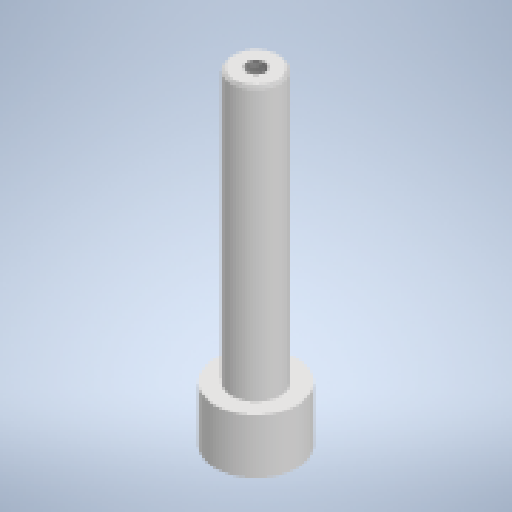
# Autodesk Inventor part: приводной вал
Saved by Autodesk Inventor 2023.2 (Build 272271030, 271C)
## iProperties
Created: 2023-08-07
Part Number: приводной вал
Material: Generic
Document SubType Name: Modeling
Designer: admin
Density: 1 g/cm^3
Appearance: Default
Author: admin
Autodesk Inventor part; units mm, degrees
ref_plane "XZ Plane" through (0, 0, 0) normal (0, 1, 0) x (-1, 0, 0)
ref_plane "XY Plane" through (0, 0, 0) normal (0, 0, 1) x (1, 0, 0)
sketch "Sketch1" plane through (0, 0, 0) normal (0, 0, 1) x (1, 0, 0)
  line L0 (0, 60) -> (0, -60)
  line L1 (0, -60) -> (15, -60)
  line L2 (9, 60) -> (0, 60)
  line L3 (9, -40) -> (15, -40)
  line L4 (9, -40) -> (9, 60)
  line L5 (15, -40) -> (15, -60)
  point P0 (0, 0)
  point P1 (0, 0)
  dimension "d17" = 18
  dimension "d18" = 20
  dimension "d19" = 30
  dimension "d42" = 100
  constraints: 13 end point, 2 horizontal, 2 midpoint, 2 perpendicular, 2 vertical, 1 coincident
  measures "d17" diameter of L4 L0
  measures "d18" distance of L3.end L1.end
  measures "d19" diameter of L5 L0
  measures "d42" distance of L3.start L2.start
revolve "Revolution1" add sketch "Sketch1" angle 360 about axis through (0, 60, 0) along (0, -1, 0)
sketch "Sketch4" plane through (0, 60, 0) normal (0, 1, 0) x (1, 0, 0)
  point P0 (0, 0)
  point P1 (0, 0)
  constraints: 1 coincident
hole "Hole1" at (0, 60, 0) direction (0, -1, 0) diameter 6.647 depth 22.2 tip angle 118 thread size "M8x1.25" class "6H" standard "ISO Metric profile"
chamfer "Chamfer1" distance 1 angle 45 1 edges at (-9, 60, 0)
ref_plane "Work Plane1" through (-9, 10, 0) normal (1, 0, 0) x (0, 1, 0)
sketch "Sketch5" plane through (-9, 10, 0) normal (1, 0, 0) x (0, 1, 0)
  line L0 (-50, 9) -> (-50, -9) projected
  line L1 (49, -9) -> (49, 9) projected
  line L2 (35, 0) -> (15, 0) construction
  line L3 (35, -3) -> (15, -3)
  line L4 (15, 3) -> (35, 3)
  arc A0 (35, -3) -> (35, 3) centre (35, 0) ccw
  arc A1 (15, 3) -> (15, -3) centre (15, 0) ccw
  line L5 (50, 8) -> (50, -8) projected
  point P0 (-10, 0)
  point P1 (25, 0)
  dimension "d36" = 6
  dimension "d37" = 20
  dimension "d39" = 15
  constraints: 8 end point, 4 point on circle, 4 tangent, 2 centre point, 1 horizontal, 1 horizontal alignment, 1 midpoint, 1 parallel
  measures "d36" distance between parallel lines of L4 L3
  measures "d37" distance of L2.start L2.end
  measures "d39" distance from line of L2.start L5
extrude "Extrusion3" cut sketch "Sketch5" along normal blind 3
body "Solid1"
